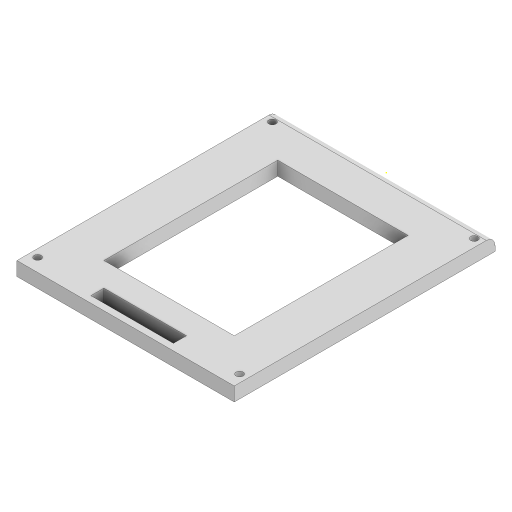
# Autodesk Inventor part: Scanner_Test_Bot
Saved by Autodesk Inventor 2023 (Build 270158000, 158)
## iProperties
Created: 2022-09-22
Part Number: Scanner_Test_Bot
Material: Generic
Document SubType Name: Modeling
Designer: Vking
Density: 1 g/cm^3
Appearance: Default
Author: Vking
Autodesk Inventor part; units mm, degrees
ref_plane "YZ Plane" through (0, 0, 0) normal (1, 0, 0) x (0, 1, 0)
ref_plane "XZ Plane" through (0, 0, 0) normal (0, 1, 0) x (-1, 0, 0)
ref_plane "XY Plane" through (0, 0, 0) normal (0, 0, 1) x (1, 0, 0)
sketch "Sketch1" plane through (0, 0, 0) normal (0, 0, 1) x (1, 0, 0)
  line L0 (-31.75, 5.08) -> (31.75, 5.08)
  line L1 (31.75, 5.08) -> (31.75, -5.08)
  line L2 (31.75, -5.08) -> (-31.75, -5.08)
  line L3 (-31.75, -5.08) -> (-31.75, 5.08)
  point P0 (0, 0)
  dimension "d0" = 63.5
  dimension "d3" = 31.75
  dimension "d4" = 10.16
  dimension "d17" = 5.08
  constraints: 8 end point, 2 parallel, 1 horizontal, 1 perpendicular
  measures "d0" distance of L0.start L0.end
  measures "d3" distance from line of L3 point (0, 0)
  measures "d4" distance of L0.end L1.end
  measures "d17" distance from line of point (0, 0) L2
extrude "Extrusion1" add sketch "Sketch1" along normal blind 76.2
sketch "Sketch3" plane through (0, 0, 76.2) normal (0, 0, 1) x (1, 0, 0)
  line L0 (-27.25, 0.3875) -> (27.25, 0.3875)
  line L1 (27.25, 0.3875) -> (27.25, -0.3745)
  line L2 (27.25, -0.3745) -> (-27.25, -0.3745)
  line L3 (-27.25, -0.3745) -> (-27.25, 0.3875)
  line L4 (-31.75, 5.08) -> (-31.75, -5.08) projected
  point P0 (0, 0)
  point P1 (-27.25, 0.0065)
  dimension "d6" = 0.762
  dimension "d7" = 54.5
  dimension "d8" = 4.5
  constraints: 8 end point, 2 parallel, 1 horizontal, 1 midpoint, 1 perpendicular
  measures "d6" distance between parallel lines of L2 L0
  measures "d7" distance of L0.start L0.end
  measures "d8" distance from line of L4 point (-27.25, 0.006)
extrude "Extrusion2" cut sketch "Sketch3" against normal blind 85.1
sketch "Sketch8" plane through (0, 0, 76.2) normal (0, 0, 1) x (1, 0, 0)
  line L0 (-31.75, 5.08) -> (-31.75, -5.08) projected
  line L1 (31.75, -5.08) -> (31.75, 5.08) projected
  line L2 (-31.75, -5.08) -> (31.75, -5.08)
  line L3 (31.75, -5.08) -> (31.75, 0.3875)
  line L4 (31.75, 0.3875) -> (-31.75, 0.3875)
  line L5 (-31.75, 0.3875) -> (-31.75, -5.08)
  line L6 (-27.25, 0.3875) -> (27.25, 0.3875) projected
  point P0 (0, 0)
  point P1 (-31.75, 0.3875)
  dimension "d30" = 0
  constraints: 8 end point, 2 parallel, 1 horizontal, 1 perpendicular, 1 point on line
  measures "d30" distance between parallel lines of L6 L4
extrude "Extrusion6" cut sketch "Sketch8" against normal blind 76.2
sketch "Sketch9" plane through (-31.75, 5.08, 0) normal (0, 1, 0) x (1, 0, 0)
  line L0 (63.5, 0) -> (0, 0) projected
  line L1 (0, 0) -> (0, -76.2) projected
  line L2 (63.5, -76.2) -> (0, -76.2) projected
  line L3 (63.5, 0) -> (63.5, -76.2) projected
  line L4 (12.7, -12.7) -> (50.8, -12.7)
  line L5 (50.8, -12.7) -> (50.8, -63.5)
  line L6 (50.8, -63.5) -> (12.7, -63.5)
  line L7 (12.7, -63.5) -> (12.7, -12.7)
  point P0 (31.75, 0)
  dimension "d33" = 12.7
  constraints: 8 end point, 3 other
  measures "d33" distance between parallel lines of L0 L4
extrude "Extrusion7" cut sketch "Sketch9" against normal blind 25.4 contours L4 L5 L6 L7
sketch "Sketch11" plane through (-31.75, 5.08, 0) normal (0, 1, 0) x (1, 0, 0)
  circle A0 centre (61.25, -72.39) radius 1.05
  line L0 (59, -76.2) -> (63.5, -76.2)
  line L1 (59, 0) -> (59, -76.2)
  circle A1 centre (2.25, -72.39) radius 1.05
  line L2 (0, 0) -> (0, -76.2)
  line L3 (0, -76.2) -> (4.5, -76.2)
  circle A2 centre (2.25, -3.81) radius 1.05
  circle A3 centre (61.25, -3.81) radius 1.05
  line L4 (4.5, 0) -> (0, 0)
  line L5 (63.5, 0) -> (59, 0)
  line L6 (50.8, -12.7) -> (50.8, -63.5) projected
  line L7 (50.8, -63.5) -> (12.7, -63.5) projected
  line L8 (12.7, -63.5) -> (12.7, -12.7) projected
  line L9 (12.7, -12.7) -> (50.8, -12.7) projected
  line L10 (63.5, 0) -> (0, 0) projected
  line L11 (0, 0) -> (0, -76.2) projected
  line L12 (63.5, -76.2) -> (0, -76.2) projected
  line L13 (63.5, 0) -> (63.5, -76.2) projected
  point P0 (31.75, -76.2)
  dimension "d37" = 2.1
  dimension "d38" = 3.81
  dimension "d39" = 2.25
  dimension "d40" = 2.25
  dimension "d41" = 2.1
  dimension "d42" = 3.81
  dimension "d43" = 2.1
  dimension "d44" = 2.1
  dimension "d45" = 3.81
  dimension "d46" = 3.81
  dimension "d47" = 2.25
  dimension "d48" = 2.25
  constraints: 12 end point, 4 centre point, 1 coincident
  measures "d37" diameter of A0
  measures "d38" distance from line of L0 A0.centre
  measures "d39" distance from line of A0.centre L1
  measures "d40" distance from line of L2 A1.centre
  measures "d41" diameter of A1
  measures "d42" distance from line of L3 A1.centre
  measures "d43" diameter of A2
  measures "d44" diameter of A3
  measures "d45" distance from line of A2.centre L4
  measures "d46" distance from line of A3.centre L5
  measures "d47" distance from line of L1 A3.centre
  measures "d48" distance from line of L2 A2.centre
extrude "Extrusion8" cut sketch "Sketch11" against normal blind 25.4 contours A0 | A1 | A2 | A3
fillet "Fillet1" radius 2.54 1 edges at (0, 5.08, 0)
sketch "Sketch13" plane through (-31.75, 5.08, 76.2) normal (0, 1, 0) x (1, 0, 0)
  point P0 (31.75, 76.2)
sketch "Sketch14" plane through (-31.75, 5.08, 76.2) normal (0, 1, 0) x (1, 0, 0)
  line L0 (19.685, 1.905) -> (43.815, 1.905)
  line L1 (43.815, 1.905) -> (43.815, 5.715)
  line L2 (43.815, 5.715) -> (19.685, 5.715)
  line L3 (19.685, 5.715) -> (19.685, 1.905)
  line L4 (63.5, 76.2) -> (0, 76.2) projected
  line L5 (0, 73.66) -> (0, 0) projected
  line L6 (63.5, 73.66) -> (63.5, 0) projected
  line L7 (63.5, 0) -> (0, 0) projected
  point P0 (31.75, 76.2)
  dimension "d54" = 1.905
  dimension "d55" = 3.81
  dimension "d61" = 24.13
  dimension "d62" = 63.5
  dimension "d63" = 19.685
  constraints: 8 end point, 2 parallel, 1 horizontal, 1 perpendicular
  measures "d54" distance between parallel lines of L7 L0
  measures "d55" distance between parallel lines of L0 L2
  measures "d61" distance of L1.end L2.end
  measures "d62" distance of L6.end L5.end
  measures "d63" distance between parallel lines of L5 L3
extrude "Extrusion9" cut sketch "Sketch14" against normal blind 25.4
sketch "Sketch15" plane through (0, 0, 0) normal (0, 0, -1) x (-1, 0, 0)
  line L0 (31.75, 0.3875) -> (-31.75, 0.3875) projected
  line L1 (-31.75, 0.3875) -> (-31.75, 5.08) projected
  line L2 (31.75, 0.3875) -> (-31.75, 0.3875)
  line L3 (-31.75, 0.3875) -> (-31.75, 1.0225)
  line L4 (-31.75, 1.0225) -> (31.75, 1.0225)
  line L5 (31.75, 1.0225) -> (31.75, 0.3875)
  point P0 (0, 0)
  dimension "d58" = 0.635
  constraints: 8 end point, 2 parallel, 1 horizontal, 1 perpendicular, 1 point on line
  measures "d58" distance between parallel lines of L0 L4
extrude "Extrusion10" cut sketch "Sketch15" against normal blind 76.2
body "Solid1"
